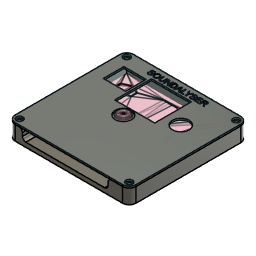
case (Autodesk Fusion 360 design; units mm, degrees)
Autodesk Fusion 360 part; units mm, degrees
sketch "Sketch1" plane through (0, 0, 0) normal (0, 1, 0) x (1, 0, 0)
sketch "Sketch1 (2)" plane through (0, 0, 0) normal (0, 1, 0) x (1, 0, 0) in component "Bottom"
  line L0 (0, 0) -> (-88.6, 0)
  line L1 (-88.6, 0) -> (-88.6, 86.3)
  line L2 (-88.6, 86.3) -> (0, 86.3)
  line L3 (0, 86.3) -> (0, 0)
  line L4 (10.5, -10.5) -> (-98.1, -10.5)
  line L5 (-98.1, -10.5) -> (-98.1, 95.8)
  line L6 (-98.1, 95.8) -> (10.5, 95.8)
  line L7 (10.5, 95.8) -> (10.5, -10.5)
  circle A0 centre (-93.1, 90.8) radius 1.7
  circle A1 centre (5.5, 90.8) radius 1.7
  circle A2 centre (-93.1, -5.5) radius 1.7
  circle A3 centre (5.5, -5.5) radius 1.7
  circle A4 centre (-93.1, 90.8) radius 3
  circle A5 centre (5.5, 90.8) radius 3
  circle A6 centre (5.5, -5.5) radius 3
  circle A7 centre (-93.1, -5.5) radius 3
  dimension "d1" = 88.6
  dimension "d2" = 86.3
  dimension "d3" = 108.6
  dimension "d4" = 106.3
  dimension "d5" = 9.5
  dimension "d6" = 9.5
  dimension "d7" = 3.4
  dimension "d8" = 5
  dimension "d9" = 5
  dimension "d10" = 3.4
  dimension "d11" = 5
  dimension "d12" = 5
  dimension "d13" = 3.4
  dimension "d14" = 5
  dimension "d15" = 5
  dimension "d16" = 3.4
  dimension "d17" = 5
  dimension "d18" = 5
  dimension "d19" = 6
  dimension "d20" = 6
  dimension "d21" = 6
  dimension "d22" = 6
  constraint horizontal L0
  constraint vertical L1
  constraint horizontal L2
  constraint vertical L3
  constraint coincident L0.start L3.end
  constraint horizontal L4
  constraint vertical L5
  constraint horizontal L6
  constraint vertical L7
  constraint concentric A0 A4
  constraint concentric A1 A5
  constraint concentric A3 A6
  constraint concentric A2 A7
  measures "d1" distance of L0.start L0.end
  measures "d2" distance of L0.start L2.end
  measures "d3" distance of L4.start L4.end
  measures "d4" distance of L4.start L6.end
  measures "d5" distance of L2 L6
  measures "d6" distance of L1 L5
  measures "d7" diameter of A0
  measures "d8" distance of L6 A0.centre
  measures "d9" distance of L5 A0.centre
  measures "d10" diameter of A1
  measures "d11" distance of L6 A1.centre
  measures "d12" distance of L7 A1.centre
  measures "d13" diameter of A2
  measures "d14" distance of L5 A2.centre
  measures "d15" distance of L4 A2.centre
  measures "d16" diameter of A3
  measures "d17" distance of L7 A3.centre
  measures "d18" distance of L4 A3.centre
  measures "d19" diameter of A4
  measures "d20" diameter of A5
  measures "d21" diameter of A6
  measures "d22" diameter of A7
extrude "Extrude1" add sketch "Sketch1 (2)" along normal blind 9.9 from surface at 3.1 contours A4 | A5 | A6 | A7 makes body 1 at (-91.7314, 9.7, -93.4696) makes body 2 at (2.7356, 9.7, -89.6347) makes body 3 at (-94.4686, 9.7, 2.8304) makes body 4 at (8.4963, 9.7, 5.6495) in component "Bottom"
extrude "Extrude2" add sketch "Sketch1 (2)" along normal blind 13 contours L4 L5 L6 L7 bodies 1 2 3 4 in component "Bottom"
extrude "Extrude3" add sketch "Sketch1 (2)" along normal blind 3 contours L0 L1 L2 L3 bodies 1 in component "Bottom"
sketch "Sketch2" plane through (0, 0, 10.5) normal (0, 0, 1) x (1, 0, 0) in component "Bottom"
  line L0 (-98.1, 0) -> (10.5, 0)
  line L1 (10.5, 0) -> (10.5, 13)
  line L2 (10.5, 13) -> (-98.1, 13)
  line L3 (-98.1, 13) -> (-98.1, 0)
sketch "Sketch4" plane through (0, 13, 0) normal (0, 1, 0) x (-1, 0, 0) in component "Bottom"
  circle A0 centre (93.1, -90.8) radius 1.7
  circle A1 centre (-5.5, 5.5) radius 1.7
  line L0 (88.6, -86.3) -> (0, -86.3)
  line L1 (0, -86.3) -> (0, 0)
  line L2 (0, 0) -> (88.6, 0)
  line L3 (88.6, 0) -> (88.6, -86.3)
  line L4 (-10.5, -95.8) -> (98.1, -95.8)
  line L5 (98.1, -95.8) -> (98.1, 10.5)
  line L6 (98.1, 10.5) -> (-10.5, 10.5)
  line L7 (-10.5, 10.5) -> (-10.5, -95.8)
  circle A2 centre (-5.5, -90.8) radius 1.7
  circle A3 centre (93.1, 5.5) radius 1.7
  line L8 (85.6, 0) -> (8.6, 0)
  line L9 (8.6, 0) -> (8.6, 10.5)
  line L10 (8.6, 10.5) -> (85.6, 10.5)
  line L11 (85.6, 10.5) -> (85.6, 0)
  line L12 (88.6, 0) -> (88.6, -86.3)
  dimension "d34" = 77
  dimension "d35" = 3
  constraint horizontal L8
  constraint vertical L9
  constraint horizontal L10
  constraint vertical L11
  constraint coincident L2 L8.start
  measures "d34" distance of L8.start L8.end
  measures "d35" distance of L11 L12
extrude "Extrude4" cut sketch "Sketch4" against normal blind 9 contours L2 L6 L8 L9 L10 L11 bodies 1 in component "Bottom"
fillet "Fillet1" radius 6 4 edges at (10.5, 6.5, -95.8) (-98.1, 6.5, -95.8) (-98.1, 6.5, 10.5) (10.5, 6.5, 10.5) on bodies 1 in component "Bottom"
fillet "Fillet2" radius 3 2 edges at (-8.6, 4, 5.25) (-85.6, 4, 5.25) on bodies 1 in component "Bottom"
fillet "Fillet3" radius 3 2 edges at (-85.6, 13, 5.25) (-8.6, 13, 5.25) on bodies 1 in component "Bottom"
other "Base Mesh Feature1" in component "Bottom"
other "Modify1" in component "Bottom"
other "Modify2" in component "Bottom"
sketch "Sketch1 (3)" plane through (0, 0, 0) normal (0, 1, 0) x (1, 0, 0) in component "Top"
  line L0 (-98.1, 95.8) -> (10.5, 95.8)
  line L1 (10.5, 95.8) -> (10.5, -10.5)
  line L2 (10.5, -10.5) -> (-98.1, -10.5)
  line L3 (-98.1, -10.5) -> (-98.1, 95.8)
  circle A0 centre (5.5, -5.5) radius 1.7
  circle A1 centre (5.5, -5.5) radius 3
  circle A2 centre (5.5, 90.8) radius 1.7
  circle A3 centre (5.5, 90.8) radius 3
  circle A4 centre (-93.1, 90.8) radius 1.7
  circle A5 centre (-93.1, 90.8) radius 3
  circle A6 centre (-93.1, -5.5) radius 1.7
  circle A7 centre (-93.1, -5.5) radius 3
  line L4 (-65, 85) -> (-29.0654, 85)
  line L5 (-29.0654, 85) -> (-29.0654, 51.9249)
  line L6 (-29.0654, 51.9249) -> (-65, 51.9249)
  line L7 (-65, 51.9249) -> (-65, 85)
  circle A8 centre (-15.7377, 62.054) radius 7.5
  line L8 (-86.8546, 81.9923) -> (-66.9162, 81.9923)
  line L9 (-66.9162, 81.9923) -> (-66.9162, 63.5467)
  line L10 (-66.9162, 63.5467) -> (-86.8546, 63.5467)
  line L11 (-86.8546, 63.5467) -> (-86.8546, 81.9923)
  circle A9 centre (-49.4302, 44.1415) radius 7.3531
  dimension "d44" = 3.4
  dimension "d45" = 6
  dimension "d46" = 3.4
  dimension "d47" = 6
  dimension "d48" = 3.4
  dimension "d49" = 6
  dimension "d50" = 3.4
  dimension "d51" = 6
  dimension "d52" = 15
  constraint horizontal L0
  constraint vertical L1
  constraint horizontal L2
  constraint vertical L3
  constraint concentric A0 A1
  constraint concentric A2 A3
  constraint concentric A4 A5
  constraint concentric A6 A7
  constraint horizontal L4
  constraint vertical L5
  constraint horizontal L6
  constraint vertical L7
  constraint horizontal L8
  constraint vertical L9
  constraint horizontal L10
  constraint vertical L11
  measures "d44" diameter of A0
  measures "d45" diameter of A1
  measures "d46" diameter of A2
  measures "d47" diameter of A3
  measures "d48" diameter of A4
  measures "d49" diameter of A5
  measures "d50" diameter of A6
  measures "d51" diameter of A7
  measures "d52" diameter of A8
extrude "Extrude1'" add sketch "Sketch1 (3)" along normal blind 1.5 separate body contours L0 L1 L2 L3 makes body 5 in component "Top"
fillet "Fillet1'" radius 6 4 edges at (10.5, 0.75, 10.5) (-98.1, 0.75, 10.5) (-98.1, 0.75, -95.8) (10.5, 0.75, -95.8) on bodies 5 in component "Top"
move_face "MoveFace1" by (0, 0, 10) 1 faces at (-45.4936, 1.5, -8.3049) on bodies 5 in component "Top"
sketch "Sketch5" plane through (0, 0, 0) normal (0, 0, 1) x (1, 0, 0) in component "Bottom"
sketch "Sketch6" plane through (0, 14.5, 0) normal (0, 1, 0) x (-1, 0, 0) in component "Bottom"
  arc A0 (-10.5, -89.8) -> (-4.5, -95.8) centre (-4.5, -89.8) ccw
  line L0 (-4.5, -95.8) -> (92.1, -95.8)
  arc A1 (92.1, -95.8) -> (98.1, -89.8) centre (92.1, -89.8) ccw
  line L1 (98.1, -89.8) -> (98.1, 4.5)
  arc A2 (98.1, 4.5) -> (92.1, 10.5) centre (92.1, 4.5) ccw
  line L2 (92.1, 10.5) -> (-4.5, 10.5)
  arc A3 (-4.5, 10.5) -> (-10.5, 4.5) centre (-4.5, 4.5) ccw
  line L3 (-10.5, 4.5) -> (-10.5, -89.8)
  circle A4 centre (93.1, 5.5) radius 3
  circle A5 centre (93.1, -90.8) radius 3
  circle A6 centre (49.4302, -44.1415) radius 7.3531
  circle A7 centre (-5.5, -90.8) radius 3
  line L4 (29.0654, -51.9249) -> (65, -51.9249)
  line L5 (65, -51.9249) -> (65, -85)
  line L6 (65, -85) -> (29.0654, -85)
  line L7 (29.0654, -85) -> (29.0654, -51.9249)
  circle A8 centre (15.7377, -62.054) radius 7.5
  line L8 (66.9162, -63.5467) -> (86.8546, -63.5467)
  line L9 (86.8546, -63.5467) -> (86.8546, -81.9923)
  line L10 (86.8546, -81.9923) -> (66.9162, -81.9923)
  line L11 (66.9162, -81.9923) -> (66.9162, -63.5467)
  circle A9 centre (-5.5, 5.5) radius 3
  line L12 (71.7172, -88.7303) -> (34.4889, -88.7303) construction
  line L13 (34.4889, -88.7303) -> (34.4889, -92.134) construction
  line L14 (34.4889, -92.134) -> (71.7172, -92.134) construction
  line L15 (71.7172, -92.134) -> (71.7172, -88.7303) construction
  dimension "d57" = 5
  text T0 "SOUNDALYSER" font "Arial" height 5 align left top in box 37.2283 x 3.4037 at (71.7172, -88.7303) x (-1, 0) y (0, -1) spacing 1 kerned
extrude "Extrude2'" cut sketch "Sketch6" against normal blind 0.7 text T0 sketch seen with x (1, 0, 0) y (0, 1, 0) z (0, 0, 1) at (0, -13, 0) bodies 5 in component "Top"
sketch "Sketch7" plane through (0, 14.5, 0) normal (0, 1, 0) x (-1, 0, 0) in component "Bottom"
  spline S0 degree 3 poles (65.9055, -87.3898) (66.0796, -87.514) (66.4285, -87.7628) (66.6413, -88.1347) (66.7479, -88.3209) knots 0 0 0 0 0.063353 0.126897 0.126897 0.126897 0.126897
  spline S1 degree 3 poles (66.7479, -88.3209) (66.8315, -88.5206) (66.9988, -88.9202) (67.0225, -89.3528) (67.0344, -89.5692) knots 0 0 0 0 0.0644 0.128919 0.128919 0.128919 0.128919
  spline S2 degree 3 poles (67.0344, -89.5692) (67.0151, -89.9522) (66.9789, -90.6688) (66.5607, -91.2485) (66.3659, -91.5184) knots 0 0 0 0 0.112225 0.210002 0.210002 0.210002 0.210002
  spline S3 degree 3 poles (66.3659, -91.5184) (66.1228, -91.7238) (65.6247, -92.1447) (64.9735, -92.1963) (64.6401, -92.2227) knots 0 0 0 0 0.093021 0.190632 0.190632 0.190632 0.190632
  spline S4 degree 3 poles (64.6401, -92.2227) (64.4168, -92.2099) (63.9779, -92.1849) (63.5848, -91.9884) (63.3918, -91.8919) knots 0 0 0 0 0.066343 0.130352 0.130352 0.130352 0.130352
  spline S5 degree 3 poles (63.3918, -91.8919) (63.2173, -91.7702) (62.8664, -91.5256) (62.652, -91.1554) (62.5443, -90.9693) knots 0 0 0 0 0.062994 0.126646 0.126646 0.126646 0.126646
  spline S6 degree 3 poles (62.5443, -90.9693) (62.4593, -90.7615) (62.2833, -90.3316) (62.2631, -89.8672) (62.2527, -89.6272) knots 0 0 0 0 0.06682 0.138262 0.138262 0.138262 0.138262
  spline S7 degree 3 poles (62.2527, -89.6272) (62.2638, -89.3837) (62.2853, -88.9116) (62.4701, -88.4769) (62.5596, -88.2664) knots 0 0 0 0 0.072457 0.140505 0.140505 0.140505 0.140505
  spline S8 degree 3 poles (62.5596, -88.2664) (62.6714, -88.0791) (62.8919, -87.7095) (63.2518, -87.4738) (63.4294, -87.3574) knots 0 0 0 0 0.064474 0.127275 0.127275 0.127275 0.127275
  spline S9 degree 3 poles (63.4294, -87.3574) (63.6211, -87.2674) (64.006, -87.0867) (64.4305, -87.0614) (64.6435, -87.0488) knots 0 0 0 0 0.062907 0.126305 0.126305 0.126305 0.126305
  spline S10 degree 3 poles (64.6435, -87.0488) (64.8706, -87.0618) (65.3154, -87.0872) (65.7116, -87.2904) (65.9055, -87.3898) knots 0 0 0 0 0.06739 0.132013 0.132013 0.132013 0.132013
  line L0 (55.7281, -91.0631) -> (55.7281, -87.134)
  line L1 (55.7281, -87.134) -> (56.3625, -87.134)
  line L2 (56.3625, -87.134) -> (56.3625, -92.134)
  line L3 (56.3625, -92.134) -> (55.6838, -92.134)
  line L4 (55.6838, -92.134) -> (53.0576, -88.2084)
  line L5 (53.0576, -88.2084) -> (53.0576, -92.134)
  line L6 (53.0576, -92.134) -> (52.4232, -92.134)
  line L7 (52.4232, -92.134) -> (52.4232, -87.134)
  line L8 (52.4232, -87.134) -> (53.1019, -87.134)
  line L9 (53.1019, -87.134) -> (55.7281, -91.0631)
  line L10 (23.5931, -89.3544) -> (23.5931, -87.134)
  line L11 (23.5931, -87.134) -> (24.2547, -87.134)
  line L12 (24.2547, -87.134) -> (24.2547, -92.134)
  line L13 (24.2547, -92.134) -> (22.0378, -92.134)
  spline S11 degree 3 poles (22.0378, -92.134) (21.8403, -92.1325) (21.4954, -92.1299) (21.1633, -92.0384) (21.0214, -91.9993) knots 0 0 0 0 0.05893 0.10291 0.10291 0.10291 0.10291
  spline S12 degree 3 poles (21.0214, -91.9993) (20.9107, -91.9448) (20.685, -91.8337) (20.5396, -91.6282) (20.4655, -91.5235) knots 0 0 0 0 0.036419 0.074214 0.074214 0.074214 0.074214
  spline S13 degree 3 poles (20.4655, -91.5235) (20.4048, -91.4063) (20.2824, -91.1697) (20.2658, -90.9039) (20.2575, -90.7698) knots 0 0 0 0 0.039142 0.078961 0.078961 0.078961 0.078961
  spline S14 degree 3 poles (20.2575, -90.7698) (20.2709, -90.6004) (20.2972, -90.2671) (20.5015, -90.0028) (20.6019, -89.8728) knots 0 0 0 0 0.049779 0.097963 0.097963 0.097963 0.097963
  spline S15 degree 3 poles (20.6019, -89.8728) (20.7425, -89.7611) (21.0545, -89.513) (21.4491, -89.4459) (21.6661, -89.4089) knots 0 0 0 0 0.053023 0.117757 0.117757 0.117757 0.117757
  spline S16 degree 3 poles (21.6661, -89.4089) (21.5872, -89.37) (21.4459, -89.3001) (21.3219, -89.203) (21.267, -89.16) knots 0 0 0 0 0.026288 0.047145 0.047145 0.047145 0.047145
  spline S17 degree 3 poles (21.267, -89.16) (21.1698, -89.0628) (20.9655, -88.8588) (20.803, -88.62) (20.7179, -88.4949) knots 0 0 0 0 0.041137 0.086417 0.086417 0.086417 0.086417
  line L14 (20.7179, -88.4949) -> (19.8482, -87.134)
  line L15 (19.8482, -87.134) -> (20.6804, -87.134)
  line L16 (20.6804, -87.134) -> (21.342, -88.1743)
  spline S18 degree 3 poles (21.342, -88.1743) (21.4285, -88.3079) (21.5804, -88.5426) (21.7475, -88.7667) (21.8195, -88.8632) knots 0 0 0 0 0.047723 0.083844 0.083844 0.083844 0.083844
  spline S19 degree 3 poles (21.8195, -88.8632) (21.876, -88.9338) (21.9754, -89.0581) (22.1011, -89.1554) (22.1555, -89.1975) knots 0 0 0 0 0.026979 0.047536 0.047536 0.047536 0.047536
  spline S20 degree 3 poles (22.1555, -89.1975) (22.2044, -89.2267) (22.2995, -89.2836) (22.4057, -89.3151) (22.4573, -89.3305) knots 0 0 0 0 0.017016 0.0331 0.0331 0.0331 0.0331
  spline S21 degree 3 poles (22.4573, -89.3305) (22.5067, -89.3374) (22.6288, -89.3545) (22.7522, -89.3544) (22.8257, -89.3544) knots 0 0 0 0 0.014944 0.036951 0.036951 0.036951 0.036951
  line L17 (22.8257, -89.3544) -> (23.5931, -89.3544)
  line L18 (38.5112, -87.7241) -> (38.5112, -87.134)
  line L19 (38.5112, -87.134) -> (41.6354, -87.134)
  line L20 (41.6354, -87.134) -> (41.6354, -92.134)
  line L21 (41.6354, -92.134) -> (40.9737, -92.134)
  line L22 (40.9737, -92.134) -> (40.9737, -87.7241)
  line L23 (40.9737, -87.7241) -> (38.5112, -87.7241)
  spline S22 degree 3 poles (32.8137, -87.2466) (32.9578, -87.3199) (33.2422, -87.4647) (33.4372, -87.7172) (33.5334, -87.8417) knots 0 0 0 0 0.047839 0.094429 0.094429 0.094429 0.094429
  spline S23 degree 3 poles (33.5334, -87.8417) (33.6101, -87.9797) (33.7657, -88.2595) (33.7937, -88.5786) (33.8079, -88.7405) knots 0 0 0 0 0.046782 0.094914 0.094914 0.094914 0.094914
  line L24 (33.8079, -88.7405) -> (33.1838, -88.795)
  spline S24 degree 3 poles (33.1838, -88.795) (33.1662, -88.6788) (33.1332, -88.4612) (33.027, -88.269) (32.9775, -88.1794) knots 0 0 0 0 0.034936 0.065388 0.065388 0.065388 0.065388
  spline S25 degree 3 poles (32.9775, -88.1794) (32.9127, -88.1017) (32.7739, -87.9353) (32.5785, -87.8409) (32.4744, -87.7906) knots 0 0 0 0 0.030005 0.064234 0.064234 0.064234 0.064234
  spline S26 degree 3 poles (32.4744, -87.7906) (32.3548, -87.7473) (32.1069, -87.6577) (31.8434, -87.6475) (31.707, -87.6422) knots 0 0 0 0 0.037908 0.078579 0.078579 0.078579 0.078579
  spline S27 degree 3 poles (31.707, -87.6422) (31.5872, -87.6459) (31.3591, -87.6529) (31.1417, -87.722) (31.0385, -87.7548) knots 0 0 0 0 0.035752 0.068081 0.068081 0.068081 0.068081
  spline S28 degree 3 poles (31.0385, -87.7548) (30.9499, -87.7933) (30.7837, -87.8656) (30.6633, -88.0005) (30.6071, -88.0634) knots 0 0 0 0 0.028587 0.053609 0.053609 0.053609 0.053609
  spline S29 degree 3 poles (30.6071, -88.0634) (30.5658, -88.1299) (30.4841, -88.2612) (30.4717, -88.4153) (30.4655, -88.4915) knots 0 0 0 0 0.023091 0.045667 0.045667 0.045667 0.045667
  spline S30 degree 3 poles (30.4655, -88.4915) (30.4708, -88.567) (30.4813, -88.7157) (30.5622, -88.8408) (30.6019, -88.9025) knots 0 0 0 0 0.022304 0.043934 0.043934 0.043934 0.043934
  spline S31 degree 3 poles (30.6019, -88.9025) (30.6595, -88.9603) (30.7884, -89.09) (30.9582, -89.1592) (31.0521, -89.1975) knots 0 0 0 0 0.024245 0.054313 0.054313 0.054313 0.054313
  spline S32 degree 3 poles (31.0521, -89.1975) (31.1596, -89.2319) (31.4527, -89.3259) (31.7524, -89.3966) (31.9423, -89.4413) knots 0 0 0 0 0.033833 0.092327 0.092327 0.092327 0.092327
  spline S33 degree 3 poles (31.9423, -89.4413) (32.1397, -89.4885) (32.4699, -89.5674) (32.782, -89.7001) (32.9075, -89.7534) knots 0 0 0 0 0.060743 0.101593 0.101593 0.101593 0.101593
  spline S34 degree 3 poles (32.9075, -89.7534) (33.0175, -89.8169) (33.2261, -89.9374) (33.3722, -90.1286) (33.4413, -90.219) knots 0 0 0 0 0.037661 0.07145 0.07145 0.07145 0.07145
  spline S35 degree 3 poles (33.4413, -90.219) (33.4925, -90.3151) (33.5963, -90.5097) (33.61, -90.7299) (33.6169, -90.8414) knots 0 0 0 0 0.032271 0.065348 0.065348 0.065348 0.065348
  spline S36 degree 3 poles (33.6169, -90.8414) (33.6076, -90.9661) (33.5888, -91.2179) (33.4647, -91.438) (33.4021, -91.5491) knots 0 0 0 0 0.037014 0.074774 0.074774 0.074774 0.074774
  spline S37 degree 3 poles (33.4021, -91.5491) (33.32, -91.6531) (33.1501, -91.8684) (32.9025, -91.9873) (32.7745, -92.0488) knots 0 0 0 0 0.0392 0.081166 0.081166 0.081166 0.081166
  spline S38 degree 3 poles (32.7745, -92.0488) (32.6306, -92.0985) (32.3335, -92.2012) (32.0192, -92.2131) (31.8571, -92.2193) knots 0 0 0 0 0.045409 0.093773 0.093773 0.093773 0.093773
  spline S39 degree 3 poles (31.8571, -92.2193) (31.681, -92.2134) (31.3451, -92.2021) (31.0276, -92.0924) (30.8765, -92.0402) knots 0 0 0 0 0.052502 0.100178 0.100178 0.100178 0.100178
  spline S40 degree 3 poles (30.8765, -92.0402) (30.7442, -91.9752) (30.4867, -91.8485) (30.3095, -91.623) (30.2234, -91.5133) knots 0 0 0 0 0.043593 0.08488 0.08488 0.08488 0.08488
  spline S41 degree 3 poles (30.2234, -91.5133) (30.156, -91.3924) (30.0191, -91.1471) (29.9917, -90.8674) (29.9778, -90.7254) knots 0 0 0 0 0.04104 0.083317 0.083317 0.083317 0.083317
  line L25 (29.9778, -90.7254) -> (30.6122, -90.6777)
  spline S42 degree 3 poles (30.6122, -90.6777) (30.636, -90.8231) (30.6809, -91.0971) (30.8698, -91.2992) (30.9584, -91.3939) knots 0 0 0 0 0.043094 0.081155 0.081155 0.081155 0.081155
  spline S43 degree 3 poles (30.9584, -91.3939) (31.0772, -91.4643) (31.3445, -91.6227) (31.6565, -91.6313) (31.8298, -91.6361) knots 0 0 0 0 0.040801 0.091768 0.091768 0.091768 0.091768
  spline S44 degree 3 poles (31.8298, -91.6361) (32.007, -91.6334) (32.3176, -91.6287) (32.5884, -91.4799) (32.7046, -91.4161) knots 0 0 0 0 0.052175 0.091411 0.091411 0.091411 0.091411
  spline S45 degree 3 poles (32.7046, -91.4161) (32.7846, -91.341) (32.9391, -91.1961) (32.9661, -90.9867) (32.9792, -90.8857) knots 0 0 0 0 0.031819 0.061404 0.061404 0.061404 0.061404
  spline S46 degree 3 poles (32.9792, -90.8857) (32.9714, -90.8002) (32.9559, -90.6306) (32.8415, -90.5047) (32.7848, -90.4424) knots 0 0 0 0 0.025033 0.049607 0.049607 0.049607 0.049607
  spline S47 degree 3 poles (32.7848, -90.4424) (32.6715, -90.3792) (32.3602, -90.2058) (32.01, -90.1325) (31.7871, -90.086) knots 0 0 0 0 0.038724 0.106441 0.106441 0.106441 0.106441
  spline S48 degree 3 poles (31.7871, -90.086) (31.5587, -90.0349) (31.1831, -89.951) (30.8219, -89.8188) (30.6804, -89.7671) knots 0 0 0 0 0.070116 0.115283 0.115283 0.115283 0.115283
  spline S49 degree 3 poles (30.6804, -89.7671) (30.5471, -89.6994) (30.2974, -89.5727) (30.119, -89.3575) (30.0358, -89.2572) knots 0 0 0 0 0.044271 0.082967 0.082967 0.082967 0.082967
  spline S50 degree 3 poles (30.0358, -89.2572) (29.9751, -89.149) (29.8512, -88.9281) (29.8356, -88.6752) (29.8277, -88.546) knots 0 0 0 0 0.036694 0.07495 0.07495 0.07495 0.07495
  spline S51 degree 3 poles (29.8277, -88.546) (29.8378, -88.4142) (29.8581, -88.1466) (29.9896, -87.9126) (30.0562, -87.794) knots 0 0 0 0 0.039172 0.079452 0.079452 0.079452 0.079452
  spline S52 degree 3 poles (30.0562, -87.794) (30.1428, -87.682) (30.3211, -87.451) (30.5796, -87.3149) (30.7128, -87.2449) knots 0 0 0 0 0.041948 0.086488 0.086488 0.086488 0.086488
  spline S53 degree 3 poles (30.7128, -87.2449) (30.8627, -87.1877) (31.1729, -87.0694) (31.5048, -87.0558) (31.6763, -87.0488) knots 0 0 0 0 0.047808 0.098905 0.098905 0.098905 0.098905
  spline S54 degree 3 poles (31.6763, -87.0488) (31.8862, -87.0541) (32.2756, -87.064) (32.644, -87.189) (32.8137, -87.2466) knots 0 0 0 0 0.062568 0.11604 0.11604 0.11604 0.11604
  line L26 (25.179, -87.7241) -> (25.179, -87.134)
  line L27 (25.179, -87.134) -> (28.9103, -87.134)
  line L28 (28.9103, -87.134) -> (28.9103, -92.134)
  line L29 (28.9103, -92.134) -> (25.295, -92.134)
  line L30 (25.295, -92.134) -> (25.295, -91.544)
  line L31 (25.295, -91.544) -> (28.2486, -91.544)
  line L32 (28.2486, -91.544) -> (28.2486, -90.0126)
  line L33 (28.2486, -90.0126) -> (25.4826, -90.0126)
  line L34 (25.4826, -90.0126) -> (25.4826, -89.426)
  line L35 (25.4826, -89.426) -> (28.2486, -89.426)
  line L36 (28.2486, -89.426) -> (28.2486, -87.7241)
  line L37 (28.2486, -87.7241) -> (25.179, -87.7241)
  line L38 (36.1715, -89.252) -> (36.1715, -87.134)
  line L39 (36.1715, -87.134) -> (36.8332, -87.134)
  line L40 (36.8332, -87.134) -> (36.8332, -89.252)
  line L41 (36.8332, -89.252) -> (38.7602, -92.134)
  line L42 (38.7602, -92.134) -> (37.9553, -92.134)
  line L43 (37.9553, -92.134) -> (36.9696, -90.6265)
  spline S55 degree 3 poles (36.9696, -90.6265) (36.8806, -90.4863) (36.7043, -90.2084) (36.5419, -89.9223) (36.4614, -89.7807) knots 0 0 0 0 0.049828 0.098689 0.098689 0.098689 0.098689
  spline S56 degree 3 poles (36.4614, -89.7807) (36.3793, -89.9202) (36.2038, -90.2186) (36.0158, -90.5093) (35.9157, -90.6641) knots 0 0 0 0 0.048563 0.103842 0.103842 0.103842 0.103842
  line L44 (35.9157, -90.6641) -> (34.9471, -92.134)
  line L45 (34.9471, -92.134) -> (34.1763, -92.134)
  line L46 (34.1763, -92.134) -> (36.1715, -89.252)
  line L47 (45.5644, -88.6484) -> (46.1135, -87.134)
  line L48 (46.1135, -87.134) -> (46.8161, -87.134)
  line L49 (46.8161, -87.134) -> (44.8959, -92.134)
  line L50 (44.8959, -92.134) -> (44.1831, -92.134)
  line L51 (44.1831, -92.134) -> (42.1367, -87.134)
  line L52 (42.1367, -87.134) -> (42.8905, -87.134)
  line L53 (42.8905, -87.134) -> (43.4737, -88.6484)
  line L54 (43.4737, -88.6484) -> (45.5644, -88.6484)
  spline S57 degree 3 poles (48.7039, -87.2193) (48.8287, -87.1945) (49.0938, -87.1417) (49.3641, -87.1367) (49.5071, -87.134) knots 0 0 0 0 0.0381 0.080914 0.080914 0.080914 0.080914
  line L55 (49.5071, -87.134) -> (51.3114, -87.134)
  line L56 (51.3114, -87.134) -> (51.3114, -92.134)
  line L57 (51.3114, -92.134) -> (49.589, -92.134)
  spline S58 degree 3 poles (49.589, -92.134) (49.4171, -92.1333) (49.1184, -92.1321) (48.8239, -92.0832) (48.6988, -92.0624) knots 0 0 0 0 0.051447 0.089431 0.089431 0.089431 0.089431
  spline S59 degree 3 poles (48.6988, -92.0624) (48.5622, -92.0239) (48.2959, -91.9489) (48.0737, -91.7844) (47.9655, -91.7043) knots 0 0 0 0 0.042175 0.082214 0.082214 0.082214 0.082214
  spline S60 degree 3 poles (47.9655, -91.7043) (47.8414, -91.5836) (47.5884, -91.3376) (47.4462, -91.0145) (47.3738, -90.8499) knots 0 0 0 0 0.051428 0.104801 0.104801 0.104801 0.104801
  spline S61 degree 3 poles (47.3738, -90.8499) (47.3166, -90.6656) (47.1966, -90.2786) (47.1842, -89.8735) (47.1777, -89.6613) knots 0 0 0 0 0.05763 0.120959 0.120959 0.120959 0.120959
  spline S62 degree 3 poles (47.1777, -89.6613) (47.1819, -89.4813) (47.1899, -89.1399) (47.2719, -88.8085) (47.3107, -88.6518) knots 0 0 0 0 0.05382 0.1021 0.1021 0.1021 0.1021
  spline S63 degree 3 poles (47.3107, -88.6518) (47.3556, -88.5151) (47.4399, -88.2584) (47.5843, -88.0302) (47.6517, -87.9236) knots 0 0 0 0 0.042972 0.080682 0.080682 0.080682 0.080682
  spline S64 degree 3 poles (47.6517, -87.9236) (47.7207, -87.834) (47.8526, -87.6627) (48.0248, -87.5323) (48.1071, -87.47) knots 0 0 0 0 0.03373 0.064527 0.064527 0.064527 0.064527
  spline S65 degree 3 poles (48.1071, -87.47) (48.1963, -87.4176) (48.384, -87.3074) (48.5939, -87.2496) (48.7039, -87.2193) knots 0 0 0 0 0.030916 0.064986 0.064986 0.064986 0.064986
  spline S66 degree 3 poles (58.4294, -87.9765) (58.3396, -88.1342) (58.1174, -88.525) (58.1184, -88.9783) (58.119, -89.2486) knots 0 0 0 0 0.053658 0.13291 0.13291 0.13291 0.13291
  line L58 (58.119, -89.2486) -> (58.119, -92.134)
  line L59 (58.119, -92.134) -> (57.4573, -92.134)
  line L60 (57.4573, -92.134) -> (57.4573, -89.2452)
  spline S67 degree 3 poles (57.4573, -89.2452) (57.4605, -89.0181) (57.4661, -88.6113) (57.5783, -88.2207) (57.6279, -88.0481) knots 0 0 0 0 0.06775 0.121395 0.121395 0.121395 0.121395
  spline S68 degree 3 poles (57.6279, -88.0481) (57.698, -87.906) (57.8423, -87.614) (58.1074, -87.4242) (58.2435, -87.3267) knots 0 0 0 0 0.046779 0.096143 0.096143 0.096143 0.096143
  spline S69 degree 3 poles (58.2435, -87.3267) (58.4121, -87.2458) (58.7805, -87.0691) (59.1898, -87.0559) (59.4116, -87.0488) knots 0 0 0 0 0.055521 0.121246 0.121246 0.121246 0.121246
  spline S70 degree 3 poles (59.4116, -87.0488) (59.6276, -87.055) (60.0261, -87.0665) (60.393, -87.2204) (60.561, -87.2909) knots 0 0 0 0 0.064151 0.118358 0.118358 0.118358 0.118358
  spline S71 degree 3 poles (60.561, -87.2909) (60.6991, -87.3802) (60.9736, -87.5577) (61.124, -87.8477) (61.1988, -87.9918) knots 0 0 0 0 0.048411 0.096232 0.096232 0.096232 0.096232
  spline S72 degree 3 poles (61.1988, -87.9918) (61.2543, -88.1715) (61.3803, -88.579) (61.3864, -89.0063) (61.3898, -89.2452) knots 0 0 0 0 0.05613 0.12736 0.12736 0.12736 0.12736
  line L61 (61.3898, -89.2452) -> (61.3898, -92.134)
  line L62 (61.3898, -92.134) -> (60.7281, -92.134)
  line L63 (60.7281, -92.134) -> (60.7281, -89.2486)
  spline S73 degree 3 poles (60.7281, -89.2486) (60.7275, -89.0587) (60.7263, -88.7332) (60.6421, -88.4193) (60.6071, -88.2885) knots 0 0 0 0 0.056655 0.097123 0.097123 0.097123 0.097123
  spline S74 degree 3 poles (60.6071, -88.2885) (60.5591, -88.1914) (60.4628, -87.9959) (60.2819, -87.874) (60.191, -87.8128) knots 0 0 0 0 0.0319 0.064192 0.064192 0.064192 0.064192
  spline S75 degree 3 poles (60.191, -87.8128) (60.0833, -87.7641) (59.8544, -87.6605) (59.6029, -87.6508) (59.4696, -87.6456) knots 0 0 0 0 0.035099 0.074671 0.074671 0.074671 0.074671
  spline S76 degree 3 poles (59.4696, -87.6456) (59.2534, -87.6505) (58.8712, -87.6591) (58.5631, -87.8804) (58.4294, -87.9765) knots 0 0 0 0 0.063045 0.111418 0.111418 0.111418 0.111418
  spline S77 degree 3 poles (70.723, -87.2466) (70.8671, -87.3199) (71.1515, -87.4647) (71.3465, -87.7172) (71.4427, -87.8417) knots 0 0 0 0 0.047839 0.094429 0.094429 0.094429 0.094429
  spline S78 degree 3 poles (71.4427, -87.8417) (71.5194, -87.9797) (71.675, -88.2595) (71.703, -88.5786) (71.7172, -88.7405) knots 0 0 0 0 0.046783 0.094914 0.094914 0.094914 0.094914
  line L64 (71.7172, -88.7405) -> (71.0931, -88.795)
  spline S79 degree 3 poles (71.0931, -88.795) (71.0755, -88.6788) (71.0425, -88.4612) (70.9362, -88.269) (70.8867, -88.1794) knots 0 0 0 0 0.034936 0.065388 0.065388 0.065388 0.065388
  spline S80 degree 3 poles (70.8867, -88.1794) (70.8219, -88.1017) (70.6832, -87.9353) (70.4878, -87.8409) (70.3837, -87.7906) knots 0 0 0 0 0.030005 0.064234 0.064234 0.064234 0.064234
  spline S81 degree 3 poles (70.3837, -87.7906) (70.2641, -87.7473) (70.0162, -87.6577) (69.7527, -87.6475) (69.6163, -87.6422) knots 0 0 0 0 0.037908 0.078579 0.078579 0.078579 0.078579
  spline S82 degree 3 poles (69.6163, -87.6422) (69.4965, -87.6459) (69.2684, -87.6529) (69.051, -87.722) (68.9478, -87.7548) knots 0 0 0 0 0.035752 0.068081 0.068081 0.068081 0.068081
  spline S83 degree 3 poles (68.9478, -87.7548) (68.8592, -87.7933) (68.693, -87.8656) (68.5726, -88.0005) (68.5163, -88.0634) knots 0 0 0 0 0.028587 0.053609 0.053609 0.053609 0.053609
  spline S84 degree 3 poles (68.5163, -88.0634) (68.475, -88.1299) (68.3934, -88.2612) (68.3809, -88.4153) (68.3748, -88.4915) knots 0 0 0 0 0.023091 0.045667 0.045667 0.045667 0.045667
  spline S85 degree 3 poles (68.3748, -88.4915) (68.3801, -88.567) (68.3906, -88.7157) (68.4714, -88.8408) (68.5112, -88.9025) knots 0 0 0 0 0.022304 0.043934 0.043934 0.043934 0.043934
  spline S86 degree 3 poles (68.5112, -88.9025) (68.5688, -88.9603) (68.6976, -89.09) (68.8674, -89.1592) (68.9614, -89.1975) knots 0 0 0 0 0.024245 0.054313 0.054313 0.054313 0.054313
  spline S87 degree 3 poles (68.9614, -89.1975) (69.0688, -89.2319) (69.362, -89.3259) (69.6617, -89.3966) (69.8516, -89.4413) knots 0 0 0 0 0.033833 0.092327 0.092327 0.092327 0.092327
  spline S88 degree 3 poles (69.8516, -89.4413) (70.049, -89.4885) (70.3792, -89.5674) (70.6913, -89.7001) (70.8168, -89.7534) knots 0 0 0 0 0.060743 0.101593 0.101593 0.101593 0.101593
  spline S89 degree 3 poles (70.8168, -89.7534) (70.9268, -89.8169) (71.1354, -89.9374) (71.2815, -90.1286) (71.3506, -90.219) knots 0 0 0 0 0.037661 0.07145 0.07145 0.07145 0.07145
  spline S90 degree 3 poles (71.3506, -90.219) (71.4018, -90.3151) (71.5055, -90.5097) (71.5193, -90.7299) (71.5262, -90.8414) knots 0 0 0 0 0.032271 0.065348 0.065348 0.065348 0.065348
  spline S91 degree 3 poles (71.5262, -90.8414) (71.5169, -90.9661) (71.4981, -91.2179) (71.374, -91.438) (71.3114, -91.5491) knots 0 0 0 0 0.037014 0.074774 0.074774 0.074774 0.074774
  spline S92 degree 3 poles (71.3114, -91.5491) (71.2293, -91.6531) (71.0593, -91.8684) (70.8118, -91.9873) (70.6838, -92.0488) knots 0 0 0 0 0.0392 0.081166 0.081166 0.081166 0.081166
  spline S93 degree 3 poles (70.6838, -92.0488) (70.5399, -92.0985) (70.2427, -92.2012) (69.9284, -92.2131) (69.7663, -92.2193) knots 0 0 0 0 0.045409 0.093773 0.093773 0.093773 0.093773
  spline S94 degree 3 poles (69.7663, -92.2193) (69.5903, -92.2134) (69.2543, -92.2021) (68.9369, -92.0924) (68.7858, -92.0402) knots 0 0 0 0 0.052502 0.100178 0.100178 0.100178 0.100178
  spline S95 degree 3 poles (68.7858, -92.0402) (68.6535, -91.9752) (68.396, -91.8485) (68.2188, -91.623) (68.1326, -91.5133) knots 0 0 0 0 0.043593 0.08488 0.08488 0.08488 0.08488
  spline S96 degree 3 poles (68.1326, -91.5133) (68.0652, -91.3924) (67.9284, -91.1471) (67.901, -90.8674) (67.8871, -90.7254) knots 0 0 0 0 0.04104 0.083317 0.083317 0.083317 0.083317
  line L65 (67.8871, -90.7254) -> (68.5214, -90.6777)
  spline S97 degree 3 poles (68.5214, -90.6777) (68.5453, -90.8231) (68.5902, -91.0971) (68.7791, -91.2992) (68.8676, -91.3939) knots 0 0 0 0 0.043094 0.081155 0.081155 0.081155 0.081155
  spline S98 degree 3 poles (68.8676, -91.3939) (68.9865, -91.4643) (69.2538, -91.6227) (69.5658, -91.6313) (69.739, -91.6361) knots 0 0 0 0 0.040802 0.091768 0.091768 0.091768 0.091768
  spline S99 degree 3 poles (69.739, -91.6361) (69.9163, -91.6334) (70.2269, -91.6287) (70.4977, -91.4799) (70.6139, -91.4161) knots 0 0 0 0 0.052175 0.091411 0.091411 0.091411 0.091411
  spline S100 degree 3 poles (70.6139, -91.4161) (70.6939, -91.341) (70.8484, -91.1961) (70.8754, -90.9867) (70.8884, -90.8857) knots 0 0 0 0 0.031819 0.061404 0.061404 0.061404 0.061404
  spline S101 degree 3 poles (70.8884, -90.8857) (70.8806, -90.8002) (70.8652, -90.6306) (70.7507, -90.5047) (70.694, -90.4424) knots 0 0 0 0 0.025033 0.049607 0.049607 0.049607 0.049607
  spline S102 degree 3 poles (70.694, -90.4424) (70.5808, -90.3792) (70.2695, -90.2058) (69.9192, -90.1325) (69.6964, -90.086) knots 0 0 0 0 0.038725 0.106441 0.106441 0.106441 0.106441
  spline S103 degree 3 poles (69.6964, -90.086) (69.468, -90.0349) (69.0924, -89.951) (68.7312, -89.8188) (68.5897, -89.7671) knots 0 0 0 0 0.070116 0.115283 0.115283 0.115283 0.115283
  spline S104 degree 3 poles (68.5897, -89.7671) (68.4564, -89.6994) (68.2067, -89.5727) (68.0283, -89.3575) (67.945, -89.2572) knots 0 0 0 0 0.044271 0.082966 0.082966 0.082966 0.082966
  spline S105 degree 3 poles (67.945, -89.2572) (67.8844, -89.149) (67.7604, -88.9281) (67.7449, -88.6752) (67.737, -88.546) knots 0 0 0 0 0.036694 0.07495 0.07495 0.07495 0.07495
  spline S106 degree 3 poles (67.737, -88.546) (67.747, -88.4142) (67.7674, -88.1466) (67.8989, -87.9126) (67.9655, -87.794) knots 0 0 0 0 0.039172 0.079452 0.079452 0.079452 0.079452
  spline S107 degree 3 poles (67.9655, -87.794) (68.052, -87.682) (68.2304, -87.451) (68.4889, -87.3149) (68.6221, -87.2449) knots 0 0 0 0 0.041948 0.086488 0.086488 0.086488 0.086488
  spline S108 degree 3 poles (68.6221, -87.2449) (68.772, -87.1877) (69.0822, -87.0694) (69.4141, -87.0558) (69.5856, -87.0488) knots 0 0 0 0 0.047808 0.098905 0.098905 0.098905 0.098905
  spline S109 degree 3 poles (69.5856, -87.0488) (69.7955, -87.0541) (70.1849, -87.064) (70.5533, -87.189) (70.723, -87.2466) knots 0 0 0 0 0.062568 0.11604 0.11604 0.11604 0.11604
  arc A0 (-10.5, -89.8) -> (-4.5, -95.8) centre (-4.5, -89.8) ccw
  line L66 (-4.5, -95.8) -> (92.1, -95.8)
  arc A1 (92.1, -95.8) -> (98.1, -89.8) centre (92.1, -89.8) ccw
  line L67 (98.1, -89.8) -> (98.1, 4.5)
  arc A2 (98.1, 4.5) -> (92.1, 10.5) centre (92.1, 4.5) ccw
  line L68 (92.1, 10.5) -> (-4.5, 10.5)
  arc A3 (-4.5, 10.5) -> (-10.5, 4.5) centre (-4.5, 4.5) ccw
  line L69 (-10.5, 4.5) -> (-10.5, -89.8)
  circle A4 centre (93.1, 5.5) radius 3
  circle A5 centre (93.1, -90.8) radius 3
  circle A6 centre (49.4302, -44.1415) radius 7.3531
  circle A7 centre (-5.5, -90.8) radius 3
  line L70 (29.0654, -51.9249) -> (65, -51.9249)
  line L71 (65, -51.9249) -> (65, -85)
  line L72 (65, -85) -> (29.0654, -85)
  line L73 (29.0654, -85) -> (29.0654, -51.9249)
  circle A8 centre (15.7377, -62.054) radius 7.5
  line L74 (66.9162, -63.5467) -> (86.8546, -63.5467)
  line L75 (86.8546, -63.5467) -> (86.8546, -81.9923)
  line L76 (86.8546, -81.9923) -> (66.9162, -81.9923)
  line L77 (66.9162, -81.9923) -> (66.9162, -63.5467)
  circle A9 centre (-5.5, 5.5) radius 3
component "Bottom" placed x (1, 0, 0) y (0, 1, 0) z (0, 0, 1) at (0, 0, 0)
component "Top" placed x (1, 0, 0) y (0, 1, 0) z (0, 0, 1) at (0, 13, 0) in component "Bottom"
